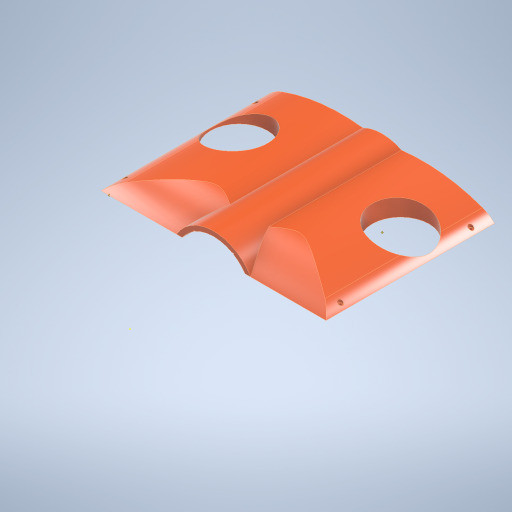
# Autodesk Inventor part: korpus3_gora
Saved by Autodesk Inventor 2024 (Build 280153000, 153)
## iProperties
Created: 2025-05-21
Part Number: korpus3_gora
Material: Tworzywo sztuczne PET
Document SubType Name: Modeling
Designer: Paweł
Density: 1.541 g/cm^3
Appearance: Gładki — jasnopomarańczowy
Mass: 287.612 g
Surface Area: 857.591 cm^2
Volume: 186.64 cm^3
Author: Paweł
Autodesk Inventor part; units mm, degrees
sketch "Szkic1" plane through (0, 0, 0) normal (0, 0, 1) x (1, 0, 0)
  arc A0 (-98.4086, -33.9749) -> (-78.2644, -32.9739) centre (-90, 0) ccw
  arc A1 (119.2902, -19.1594) -> (125, 0) centre (90, 0) ccw
  arc A2 (19.3649, -35) -> (103.6215, -25.7743) centre (42.8262, 140.0954) ccw
  arc A3 (103.6215, -25.7743) -> (125, 0) centre (91.4189, 6.1005) ccw
  line L0 (0, 31.2952) -> (0, 40)
  arc A4 (-103.6215, -25.7743) -> (-19.3649, -35) centre (-42.8262, 140.0954) ccw
  arc A5 (-125, 0) -> (-103.6215, -25.7743) centre (-91.4189, 6.1005) ccw
  arc A6 (-19.3649, 35) -> (-103.6215, 25.7743) centre (-42.8262, -140.0954) ccw
  arc A7 (-103.6215, 25.7743) -> (-125, 0) centre (-91.4189, -6.1005) ccw
  arc A8 (-19.3649, -35) -> (19.3649, -35) centre (0, 0) ccw
  arc A9 (19.3649, 35) -> (-19.3649, 35) centre (0, 0) ccw
  arc A10 (105.3748, -30.457) -> (130.0712, 0) centre (91.4189, 6.1005) ccw
  arc A11 (20.2973, -40.1624) -> (105.3748, -30.457) centre (42.8262, 140.0954) ccw
  arc A12 (-20.2973, -40.1624) -> (20.2973, -40.1624) centre (0, 0) ccw
  arc A13 (-105.3748, -30.457) -> (-20.2973, -40.1624) centre (-42.8262, 140.0954) ccw
  arc A14 (-130.0712, 0) -> (-105.3748, -30.457) centre (-91.4189, 6.1005) ccw
  arc A15 (-105.3748, 30.457) -> (-130.0712, 0) centre (-91.4189, -6.1005) ccw
  arc A16 (-20.2973, 40.1624) -> (-105.3748, 30.457) centre (-42.8262, -140.0954) ccw
  arc A17 (20.2973, 40.1624) -> (-20.2973, 40.1624) centre (0, 0) ccw
  line L1 (0, 0) -> (0, 40)
  arc A18 (103.6215, 25.7743) -> (19.3649, 35) centre (42.8262, -140.0954) ccw
  arc A19 (125, 0) -> (103.6215, 25.7743) centre (91.4189, -6.1005) ccw
  arc A20 (130.0712, 0) -> (105.3748, 30.457) centre (91.4189, -6.1005) ccw
  arc A21 (105.3748, 30.457) -> (20.2973, 40.1624) centre (42.8262, -140.0954) ccw
  point P0 (-119.2902, -19.1594)
  dimension "d1" = 70
  dimension "d2" = 70
  dimension "d4" = 250
  dimension "d6" = 90
  constraints: 46 point on circle, 22 centre point, 10 symmetric about line, 4 end point, 2 horizontal alignment, 1 coincident, 1 collinear, 1 vertical, 13 other
  measures "d1" diameter of A1
  measures "d2" diameter of A0
  measures "d6" distance of point (0, 0) A0.centre
extrude "Wyciągnięcie proste1" add sketch "Szkic1" along normal blind 130 and the other way blind 130
sketch "Szkic2" plane through (0, 0, 130) normal (0, 0, 1) x (1, 0, 0)
  arc A0 (-20.2973, 40.1624) -> (-105.3748, 30.457) centre (-42.8262, -140.0954) ccw projected
  arc A1 (-105.3748, 30.457) -> (-130.0712, 0) centre (-91.4189, -6.1005) ccw projected
  arc A2 (-130.0712, 0) -> (-105.3748, -30.457) centre (-91.4189, 6.1005) ccw projected
  arc A3 (-105.3748, -30.457) -> (-20.2973, -40.1624) centre (-42.8262, 140.0954) ccw projected
  arc A4 (-20.2973, -40.1624) -> (20.2973, -40.1624) centre (0, 0) ccw projected
  arc A5 (20.2973, -40.1624) -> (105.3748, -30.457) centre (42.8262, 140.0954) ccw projected
  arc A6 (105.3748, -30.457) -> (130.0712, 0) centre (91.4189, 6.1005) ccw projected
  arc A7 (130.0712, 0) -> (105.3748, 30.457) centre (91.4189, -6.1005) ccw projected
  arc A8 (105.3748, 30.457) -> (20.2973, 40.1624) centre (42.8262, -140.0954) ccw projected
  arc A9 (20.2973, 40.1624) -> (-20.2973, 40.1624) centre (0, 0) ccw projected
extrude "Wyciągnięcie proste2" add sketch "Szkic2" along normal mid plane 10
sketch "Szkic8" plane through (0, 0, 135) normal (0, 0, 1) x (1, 0, 0)
  circle A0 centre (0, 0) radius 45
  circle A1 centre (0, 0) radius 40
  constraints: 2 centre point, 2 coincident
extrude "Wyciągnięcie proste3" add sketch "Szkic8" along normal blind 70 contours A0 | A1
sketch "Szkic18" plane through (0, 0, 205) normal (0, 0, 1) x (1, 0, 0)
  circle A0 centre (0, 0) radius 45 projected
extrude "Wyciągnięcie proste11" add sketch "Szkic18" along normal blind 5
sketch "Szkic7" plane through (0, 0, 135) normal (0, 0, 1) x (1, 0, 0)
  point P0 (0, 0)
sketch "Szkic10" plane through (0, 0, 205) normal (0, 0, 1) x (1, 0, 0)
  circle A0 centre (0, 0) radius 45 projected
  circle A1 centre (0, 0) radius 40
  dimension "d59" = 5
  constraints: 1 centre point
  measures "d59" radial gap between concentric circles of A0 A1
extrude "Wyciągnięcie proste10" cut sketch "Szkic10" against normal blind 126.25 contours A1
sketch "Szkic12" plane through (0, 0, 0) normal (0, 1, 0) x (-1, 0, 0)
  circle A0 centre (85.2973, -65) radius 32.5
  line L0 (20.2973, -130) -> (20.2973, 135) projected
  line L1 (20.2973, -130) -> (105.3748, -130) projected
  circle A1 centre (-84.3649, -65) radius 32.5
  line L2 (-19.3649, -130) -> (-19.3649, 125) projected
  line L3 (-19.3649, -130) -> (-103.6215, -130) projected
  circle A2 centre (0, 150) radius 32.5
  line L4 (45, 205) -> (-45, 205) projected
  point P0 (0, 0)
  point P1 (-19.3649, 130)
  dimension "d37" = 65
  dimension "d38" = 65
  dimension "d39" = 65
  dimension "d49" = 65
  dimension "d50" = 65
  dimension "d51" = 65
  dimension "d54" = 65
  dimension "d55" = 55
  constraints: 3 centre point
  measures "d37" diameter of A0
  measures "d38" distance from line of L0 A0.centre
  measures "d39" distance from line of L1 A0.centre
  measures "d49" diameter of A1
  measures "d50" distance from line of L2 A1.centre
  measures "d51" distance from line of L3 A1.centre
  measures "d54" diameter of A2
  measures "d55" distance from line of A2.centre L4
extrude "Wyciągnięcie proste6" add sketch "Szkic12" along normal mid plane 111.25
sketch "Szkic33" plane through (84.3649, 55.625, -65) normal (0, 1, 0) x (1, 0, 0)
  circle A0 centre (-84.3649, -215) radius 32.5 projected
  circle A1 centre (0, 0) radius 32.5 projected
  circle A2 centre (-169.6622, 0) radius 32.5 projected
  circle A3 centre (0, 0) radius 30
  circle A4 centre (-169.6622, 0) radius 30
  circle A5 centre (-84.3649, -215) radius 30
  line L0 (-129.3649, -275) -> (-39.3649, -275) projected
  point P0 (-84.3649, -65)
  dimension "d106" = 60
  dimension "d107" = 60
  dimension "d108" = 60
  dimension "d224" = 60
  constraints: 3 centre point, 3 coincident
  measures "d106" diameter of A3
  measures "d107" diameter of A4
  measures "d108" diameter of A5
  measures "d224" distance from line of L0 A0.centre
extrude "Wyciągnięcie proste20" cut sketch "Szkic33" against normal blind 159.75 contours A3 | A4 | A5
sketch "Szkic34" plane through (0, 0, -130) normal (0, 0, -1) x (-1, 0, 0)
  arc A0 (-20.2973, -40.1624) -> (20.2973, -40.1624) centre (0, 0) ccw projected
  arc A1 (20.2973, -40.1624) -> (105.3748, -30.457) centre (42.8262, 140.0954) ccw projected
  arc A2 (105.3748, -30.457) -> (130.0712, 0) centre (91.4189, 6.1005) ccw projected
  arc A3 (130.0712, 0) -> (105.3748, 30.457) centre (91.4189, -6.1005) ccw projected
  arc A4 (105.3748, 30.457) -> (20.2973, 40.1624) centre (42.8262, -140.0954) ccw projected
  arc A5 (20.2973, 40.1624) -> (-20.2973, 40.1624) centre (0, 0) ccw projected
  arc A6 (-20.2973, 40.1624) -> (-105.3748, 30.457) centre (-42.8262, -140.0954) ccw projected
  arc A7 (-105.3748, 30.457) -> (-130.0712, 0) centre (-91.4189, -6.1005) ccw projected
  arc A8 (-130.0712, 0) -> (-105.3748, -30.457) centre (-91.4189, 6.1005) ccw projected
  arc A9 (-105.3748, -30.457) -> (-20.2973, -40.1624) centre (-42.8262, 140.0954) ccw projected
  arc A10 (19.3649, -35) -> (103.6215, -25.7743) centre (42.8262, 140.0954) ccw projected
  arc A11 (-19.3649, -35) -> (19.3649, -35) centre (0, 0) ccw projected
  arc A12 (-103.6215, -25.7743) -> (-19.3649, -35) centre (-42.8262, 140.0954) ccw projected
  arc A13 (-125, 0) -> (-103.6215, -25.7743) centre (-91.4189, 6.1005) ccw projected
  arc A14 (-103.6215, 25.7743) -> (-125, 0) centre (-91.4189, -6.1005) ccw projected
  arc A15 (-19.3649, 35) -> (-103.6215, 25.7743) centre (-42.8262, -140.0954) ccw projected
  arc A16 (19.3649, 35) -> (-19.3649, 35) centre (0, 0) ccw projected
  arc A17 (103.6215, 25.7743) -> (19.3649, 35) centre (42.8262, -140.0954) ccw projected
  arc A18 (125, 0) -> (103.6215, 25.7743) centre (91.4189, -6.1005) ccw projected
  arc A19 (103.6215, -25.7743) -> (125, 0) centre (91.4189, 6.1005) ccw projected
  arc A20 (-27.4304, 93.4644) -> (-123.6952, 79.5576) centre (-42.8262, -140.0954) ccw
  arc A21 (27.4304, 93.4644) -> (-27.4304, 93.4644) centre (0, 0) ccw
  arc A22 (123.6952, 79.5576) -> (27.4304, 93.4644) centre (42.8262, -140.0954) ccw
  arc A23 (182.7526, 0) -> (123.6952, 79.5576) centre (91.4189, -6.1005) ccw
  arc A24 (123.6952, -79.5576) -> (182.7526, 0) centre (91.4189, 6.1005) ccw
  arc A25 (27.4304, -93.4644) -> (123.6952, -79.5576) centre (42.8262, 140.0954) ccw
  arc A26 (-27.4304, -93.4644) -> (27.4304, -93.4644) centre (0, 0) ccw
  arc A27 (-123.6952, -79.5576) -> (-27.4304, -93.4644) centre (-42.8262, 140.0954) ccw
  arc A28 (-182.7526, 0) -> (-123.6952, -79.5576) centre (-91.4189, 6.1005) ccw
  arc A29 (-123.6952, 79.5576) -> (-182.7526, 0) centre (-91.4189, -6.1005) ccw
  constraints: 20 point on circle, 10 centre point, 9 other
extrude "Wyciągnięcie proste21" cut sketch "Szkic34" against normal up to surface (265 mm away) contours A21 A22 A23 A24 A25 A26 A27 A28 A29 A20
sketch "Szkic35" plane through (0, 0, 210) normal (0, 0, 1) x (1, 0, 0)
  circle A0 centre (0, 0) radius 45 projected
  circle A1 centre (0, 0) radius 93.775
  constraints: 1 centre point
extrude "Wyciągnięcie proste22" cut sketch "Szkic35" against normal up to surface (75 mm away)
ref_plane "Płaszczyzna konstrukcyjna8" through (-135.75, 0, 0) normal (1, 0, 0) x (0, 1, 0)
ref_plane "Płaszczyzna konstrukcyjna10" through (-85, 0, 0) normal (1, 0, 0) x (0, 1, 0)
ref_plane "Płaszczyzna konstrukcyjna11" through (-166.25, 0, 0) normal (1, 0, 0) x (0, 1, 0)
sketch "Szkic63" plane through (0, 0, 210) normal (0, 0, 1) x (1, 0, 0)
  circle A0 centre (0, 0) radius 45 projected
extrude "Wyciągnięcie proste37" cut sketch "Szkic63" against normal blind 16.75
ref_plane "Płaszczyzna konstrukcyjna12" through (137, 0, 0) normal (1, 0, 0) x (0, 1, 0)
sketch "Szkic64" plane through (137, 0, 0) normal (1, 0, 0) x (0, 1, 0)
  line L0 (35, -130) -> (35, 123.8992) projected
  line L1 (41.5648, -130) -> (41.5648, 135) projected
  line L2 (0, 135) -> (-30.457, 135) projected
  line L3 (-30.457, 135) -> (-41.5648, 135) projected
  line L4 (41.5648, 135) -> (30.457, 135) projected
  line L5 (30.457, 135) -> (0, 135) projected
  line L6 (2.5, 135) -> (2.5, 125)
  line L7 (-2.5, 135) -> (-2.5, 125)
  line L8 (-41.5648, -130) -> (-41.5648, 135) projected
  line L9 (-30.457, -130) -> (0, -130) projected
  line L10 (0, -130) -> (30.457, -130) projected
  line L11 (36.9405, -94.989) -> (22.5717, -94.989)
  line L12 (41.5648, -0.011) -> (-41.5648, -0.011)
  line L13 (36.9405, -35.011) -> (26.2553, -35.011)
  arc A0 (41.5648, -0.011) -> (22.5717, 47) centre (-46.3041, -8.169) ccw
  arc A1 (2.5, 125) -> (22.5717, 47) centre (167.412, 125.8543) ccw
  line L14 (0, 135) -> (0, -0.011)
  arc A2 (-22.5717, 47) -> (-41.5648, -0.011) centre (46.3041, -8.169) ccw
  arc A3 (-22.5717, 47) -> (-2.5, 125) centre (-167.412, 125.8543) ccw
  line L15 (-2.5, 135) -> (-2.5, 124.9871)
  arc A4 (-2.5, 124.9871) -> (18.3975, 44.2117) centre (167.412, 125.8543) ccw
  arc A5 (35.8963, 4.989) -> (18.3975, 44.2117) centre (-46.3041, -8.169) ccw
  line L16 (35.8963, 4.989) -> (-35.8963, 4.989)
  arc A6 (-18.3975, 44.2117) -> (-35.8963, 4.989) centre (46.3041, -8.169) ccw
  arc A7 (-18.3975, 44.2117) -> (2.5, 124.9871) centre (-167.412, 125.8543) ccw
  line L17 (2.5, 124.9871) -> (2.5, 135)
  line L18 (22.5717, 47) -> (16.9034, 47)
  line L19 (35.8963, 4.989) -> (35.8963, -0.011)
  line L20 (-22.5717, 47) -> (-16.9034, 47)
  line L21 (-35.8963, 4.989) -> (-35.8963, -0.011)
  point P0 (35, 125)
  point P1 (-40.1624, 135)
  point P2 (40.1624, 135)
  point P3 (10.9431, 47)
  dimension "d234" = 10
  dimension "d235" = 10
  dimension "d238" = 35
  dimension "d246" = 5
  constraints: 26 end point, 18 point on circle, 8 centre point, 7 point on line, 4 perpendicular, 3 symmetric about line, 2 horizontal, 2 vertical, 1 midpoint, 11 other
  measures "d234" distance of L6.start L6.end
  measures "d235" distance of L7.start L7.end
  measures "d238" distance between parallel lines of L13 L12
  measures "d246" radial gap between concentric circles of A0 A5
extrude "Wyciągnięcie proste38" cut sketch "Szkic64" against normal up to surface contours A0 A1 L6 L5 L4 L1 | L8 L3 L2 L7 A3 A2 round surface about axis through (0, 0, 0) along (0, 0, 1) radius 45 far side no
ref_plane "Płaszczyzna konstrukcyjna13" through (-136, 0, 0) normal (1, 0, 0) x (0, 1, 0)
sketch "Szkic65" plane through (-136, 0, 0) normal (1, 0, 0) x (0, 1, 0)
  arc A0 (41.5648, 0) -> (22.5717, 47.011) centre (-46.3041, -8.158) ccw
  arc A1 (2.5, 125.011) -> (22.5717, 47.011) centre (167.412, 125.8652) ccw
  arc A2 (-22.5717, 47.011) -> (-2.5, 125.011) centre (-167.412, 125.8652) ccw
  arc A3 (-22.5717, 47.011) -> (-41.5648, 0) centre (46.3041, -8.158) ccw
  line L0 (41.5648, 0) -> (-41.5648, 0)
  line L1 (2.5, 125) -> (2.5, 135) projected
  line L2 (2.5, 125.011) -> (2.5, 135)
  line L3 (2.5, 135) -> (-2.5, 135)
  line L4 (-40.1624, 135) -> (40.1624, 135) projected
  line L5 (-2.5, 125.011) -> (-2.5, 135)
  line L6 (41.5648, 0) -> (41.5648, 135)
  line L7 (41.5648, -130) -> (41.5648, 135) projected
  line L8 (-41.5648, 135) -> (-41.5648, 0)
  line L9 (-45, -130) -> (-45, 193.25) projected
  line L10 (-41.5648, 135) -> (-40.1624, 135)
  line L11 (40.1624, -130) -> (40.1624, 127.9088) projected
  line L12 (41.5648, 135) -> (30.457, 135) projected
  line L13 (40.1624, 135) -> (41.5648, 135)
  arc A4 (-18.6693, 43.8851) -> (-36.5862, -0.4622) centre (46.3041, -8.158) ccw
  arc A5 (36.5862, -0.4622) -> (18.6693, 43.8851) centre (-46.3041, -8.158) ccw
  line L14 (22.5717, 47.011) -> (16.037, 47.011)
  line L15 (-22.5717, 47.011) -> (-16.037, 47.011)
  arc A6 (18.6693, 43.8851) -> (16.037, 47.011) centre (-46.3041, -8.158) ccw
  arc A7 (-16.037, 47.011) -> (-18.6693, 43.8851) centre (46.3041, -8.158) ccw
  point P0 (0, 0)
  point P1 (-22.5717, 47.011)
  point P2 (22.5717, 47.011)
  point P3 (24.9631, 43.8851)
  point P4 (-24.9631, 43.8851)
  point P5 (-36.542, 0)
  point P6 (36.542, 0)
  point P7 (-22.5717, 47.011)
  point P8 (22.5717, 47.011)
  point P9 (-36.7423, 135)
  point P10 (36.7423, 135)
  dimension "d251" = 5
  dimension "d252" = 5
  constraints: 20 end point, 19 point on circle, 8 centre point, 3 horizontal, 3 point on line, 2 collinear, 1 concentric, 1 parallel, 1 perpendicular, 1 vertical
  measures "d251" radial gap between concentric circles of A3 A4
  measures "d252" radial gap between concentric circles of A0 A5
extrude "Wyciągnięcie proste39" cut sketch "Szkic65" along normal up to surface contours A0 A1 L1 L4 L12 L6 | L8 L10 L4 L5 A2 A3 round surface about axis through (0, 0, 0) along (0, 0, 1) radius 45 far side no
sketch "Szkic66" plane through (0, 0, 125) normal (0, 0, -1) x (-1, 0, 0)
  arc A0 (-44.9305, -2.5) -> (-27.1726, -35.8699) centre (0, 0) ccw projected
  arc A1 (-27.1726, -35.8699) -> (-20.7666, -35.1821) centre (-42.8262, 140.0954) ccw projected
  arc A2 (-20.7666, 34.187) -> (-20.7666, -34.187) centre (0, 0) ccw projected
  arc A3 (-20.7666, 35.1821) -> (-27.1726, 35.8699) centre (-42.8262, -140.0954) ccw projected
  arc A4 (-27.1726, 35.8699) -> (-44.9305, 2.5) centre (0, 0) ccw projected
  line L0 (-44.9305, 2.5) -> (-124.4483, 2.5) projected
  arc A5 (-124.4483, 2.5) -> (-125, 0) centre (-91.4189, -6.1005) ccw projected
  arc A6 (-125, 0) -> (-124.4483, -2.5) centre (-91.4189, 6.1005) ccw projected
  line L1 (-124.4483, -2.5) -> (-44.9305, -2.5) projected
  arc A7 (27.1726, -35.8699) -> (44.9305, -2.5001) centre (0, 0) ccw projected
  line L2 (44.9305, -2.5001) -> (124.4482, -2.5001) projected
  arc A8 (124.4482, -2.5001) -> (125, 0) centre (91.4189, 6.1005) ccw projected
  arc A9 (125, 0) -> (124.4482, 2.5001) centre (91.4189, -6.1005) ccw projected
  line L3 (124.4482, 2.5001) -> (44.9305, 2.5001) projected
  arc A10 (44.9305, 2.5001) -> (27.1726, 35.8699) centre (0, 0) ccw projected
  arc A11 (27.1726, 35.8699) -> (20.7666, 35.1821) centre (42.8262, -140.0954) ccw projected
  arc A12 (20.7666, -34.187) -> (20.7666, 34.187) centre (0, 0) ccw projected
  arc A13 (20.7666, -35.1821) -> (27.1726, -35.8699) centre (42.8262, 140.0954) ccw projected
  arc A14 (44.9305, -2.5) -> (44.9305, 2.5) centre (0, 0) ccw projected
  circle A15 centre (0, 0) radius 45
  line L4 (20.7666, 35.1821) -> (20.7666, 34.187) projected
  line L5 (20.7666, -34.187) -> (20.7666, -35.1821) projected
  line L6 (-20.7666, -35.1821) -> (-20.7666, -34.187) projected
  line L7 (-20.7666, 34.187) -> (-20.7666, 35.1821) projected
  point P0 (44.9305, -2.5001)
  point P1 (44.9305, -2.5)
  point P2 (-44.9305, 2.5)
  point P3 (27.1726, 35.8699)
  point P4 (27.1726, -35.8699)
  point P5 (-27.1726, 35.8699)
  point P6 (-27.1726, -35.8699)
  constraints: 1 coincident, 3 other
extrude "Wyciągnięcie proste40" add sketch "Szkic66" along normal blind 105 contours A15 A4 A3 L7 A2 L6 A1 A0 | A13 L5 A12 L4 A11 A10 A14 A7
extrude "Wyciągnięcie proste41" add sketch "Szkic64" against normal up to surface contours L19 A5 L0 A0 L12 | A5 A4 L18 A0 L0 | L12 A2 L20 A7 A6 L21 round surface about axis through (0, 0, 0) along (0, 0, 1) radius 45 far side no
extrude "Wyciągnięcie proste43" add sketch "Szkic65" along normal up to surface contours L0 L11 A0 | L11 L0 A5 A6 L14 A0 | L0 A3 L15 A7 A4 round surface about axis through (0, 0, 0) along (0, 0, 1) radius 45 far side no
ref_plane "Płaszczyzna konstrukcyjna14" through (41.7046, -16.9034, 47) normal (0, 0, 1) x (1, 0, 0)
sketch "Szkic67" plane through (41.7046, -16.9034, 47) normal (0, 0, 1) x (1, 0, 0)
  arc A0 (-21.4073, 57.0658) -> (-24.4603, 58.4682) centre (-41.7046, 16.9034) ccw projected
  arc A1 (-21.4073, 57.0658) -> (-62.0019, 57.0658) centre (-41.7046, 16.9034) ccw projected
  line L0 (-62.0019, 57.0658) -> (-62.0019, 57.0658) projected
  arc A2 (-73.3068, 48.9393) -> (-73.3068, -15.1325) centre (-41.7046, 16.9034) ccw projected
  arc A3 (-62.0019, -23.259) -> (-21.4073, -23.259) centre (-41.7046, 16.9034) ccw projected
  arc A4 (-24.4603, -24.6614) -> (-21.4073, -23.259) centre (-41.7046, 16.9034) ccw projected
  arc A5 (-2.775, -5.6684) -> (0, 0) centre (-41.7046, 16.9034) ccw projected
  arc A6 (-10.0984, -15.1286) -> (-10.0984, 48.9354) centre (-41.7046, 16.9034) ccw projected
  arc A7 (0, 33.8068) -> (-2.775, 39.4751) centre (-41.7046, 16.9034) ccw projected
  line L1 (-86.6351, 19.4034) -> (-86.6351, 19.4034) projected
  arc A8 (-86.6351, 19.4034) -> (-86.6351, 14.4034) centre (-41.7046, 16.9034) ccw projected
  line L2 (-86.6351, 14.4033) -> (-86.6351, 14.4034) projected
  arc A9 (-86.6351, 19.4034) -> (-86.6351, 14.4033) centre (-41.7046, 16.9034) ccw projected
  arc A10 (3.2259, 14.4034) -> (3.2259, 19.4034) centre (-41.7046, 16.9034) ccw projected
  arc A11 (3.2259, 14.4034) -> (3.2259, 19.4034) centre (-41.7046, 16.9034) ccw projected
  circle A12 centre (-41.7046, 16.9034) radius 45 projected
  line L3 (74.9279, 0) -> (0, 0) projected
  line L4 (74.9279, 33.8068) -> (0, 33.8068) projected
  line L5 (68.2294, 39.4751) -> (-2.775, 39.4751) projected
  line L6 (68.2294, -5.6684) -> (-2.775, -5.6684) projected
  spline S0 degree 8 poles (61.9169, -8.8709) (63.6085, -8.2233) (65.223, -7.4876) (66.7628, -6.6721) (68.2309, -5.7826) (69.6315, -4.8225) (70.9701, -3.7914) (72.2516, -2.6847) (73.4789, -1.4941) knots 0 0 0 0 0 0 0 0 0 1 1 1 1 1 1 1 1 1 projected
  spline S1 degree 4 poles (73.4789, -1.4941) (73.8652, -1.1194) (74.2349, -0.745) (74.5889, -0.3716) (74.9279, 0) knots 0 0 0 0 0 1 1 1 1 1 projected
  arc A13 (68.2294, -5.6684) -> (74.9279, 0) centre (49.7143, 23.0038) ccw projected
  spline S2 degree 8 poles (68.2294, -5.6684) (69.6364, -4.7598) (70.9108, -3.825) (72.0633, -2.8799) (73.1046, -1.9365) (74.0451, -1.0038) (74.8947, -0.0887) (75.6624, 0.804) (77.0847, 2.5803) (77.7326, 3.4621) (78.3092, 4.312) (78.8227, 5.127) (79.2802, 5.9055) (79.6881, 6.6464) (80.0521, 7.3492) (81.142, 9.5785) (81.6905, 10.9319) (82.0822, 12.0632) (82.3584, 12.9712) (82.5486, 13.6577) (82.6712, 14.1252) (82.736, 14.3742) (82.7436, 14.4034) knots 0 0 0 0 0 0 0 0 0 0.221338 0.221338 0.221338 0.221338 0.221338 0.221338 0.221338 0.453504 0.453504 0.453504 0.453504 0.453504 0.453504 0.453504 1 1 1 1 1 1 1 1 1 projected
  arc A14 (82.7436, 14.4034) -> (83.2954, 16.9034) centre (49.7143, 23.0038) ccw projected
  arc A15 (61.9169, -8.8709) -> (83.2954, 16.9034) centre (49.7143, 23.0038) ccw projected
  arc A16 (74.9279, 33.8068) -> (68.2294, 39.4751) centre (49.7143, 10.8029) ccw projected
  arc A17 (83.2954, 16.9034) -> (61.9169, 42.6777) centre (49.7143, 10.8029) ccw projected
  arc A18 (83.2954, 16.9034) -> (82.7436, 19.4034) centre (49.7143, 10.8029) ccw projected
  arc A19 (-62.0019, -23.259) -> (-58.9489, -24.6614) centre (-41.7046, 16.9034) ccw projected
  arc A20 (-58.9489, 58.4682) -> (-62.0019, 57.0658) centre (-41.7046, 16.9034) ccw projected
  arc A21 (-79.1458, 41.8665) -> (-82.6492, 35.5727) centre (-41.7046, 16.9034) ccw projected
  arc A22 (-82.6492, -1.7659) -> (-79.1458, -8.0597) centre (-41.7046, 16.9034) ccw projected
  arc A23 (-156.6047, -1.7659) -> (-147.2643, -8.0597) centre (-133.1235, 23.0038) ccw projected
  line L7 (-147.2643, -8.0597) -> (-79.1458, -8.0597) projected
  arc A24 (-82.6492, -1.7659) -> (-79.1458, -8.0597) centre (-41.7046, 16.9034) ccw projected
  line L8 (-156.6047, -1.7659) -> (-82.6492, -1.7659) projected
  arc A25 (-147.2643, 41.8665) -> (-156.6047, 35.5727) centre (-133.1235, 10.8029) ccw
  line L9 (-156.6047, 35.5727) -> (-82.6492, 35.5727)
  arc A26 (-79.1458, 41.8665) -> (-82.6492, 35.5727) centre (-41.7046, 16.9034) ccw
  line L10 (-147.2643, 41.8665) -> (-79.1458, 41.8665)
  arc A27 (-62.0019, -23.259) -> (-58.9489, -24.6614) centre (-41.7046, 16.9034) ccw projected
  arc A28 (-62.0019, -23.259) -> (-21.4073, -23.259) centre (-41.7046, 16.9034) ccw projected
  arc A29 (-24.4603, -24.6614) -> (-21.4073, -23.259) centre (-41.7046, 16.9034) ccw projected
  arc A30 (-2.775, -5.6684) -> (0, 0) centre (-41.7046, 16.9034) ccw projected
  arc A31 (-10.0984, -15.1286) -> (-10.0984, 48.9354) centre (-41.7046, 16.9034) ccw projected
  arc A32 (0, 33.8068) -> (-2.775, 39.4751) centre (-41.7046, 16.9034) ccw projected
  arc A33 (-21.4073, 57.0658) -> (-24.4603, 58.4682) centre (-41.7046, 16.9034) ccw projected
  arc A34 (-21.4073, 57.0658) -> (-62.0019, 57.0658) centre (-41.7046, 16.9034) ccw projected
  arc A35 (-58.9489, 58.4682) -> (-62.0019, 57.0658) centre (-41.7046, 16.9034) ccw projected
  arc A36 (-79.1458, 41.8665) -> (-82.6492, 35.5727) centre (-41.7046, 16.9034) ccw projected
  arc A37 (-73.3068, 48.9393) -> (-73.3068, -15.1325) centre (-41.7046, 16.9034) ccw projected
  arc A38 (-82.6492, -1.7659) -> (-79.1458, -8.0597) centre (-41.7046, 16.9034) ccw projected
  line L11 (-86.6351, 19.4034) -> (-86.6351, 19.4034) projected
  arc A39 (-86.6351, 19.4034) -> (-86.6351, 14.4034) centre (-41.7046, 16.9034) ccw projected
  line L12 (-86.6351, 14.4033) -> (-86.6351, 14.4034) projected
  arc A40 (-86.6351, 19.4034) -> (-86.6351, 14.4033) centre (-41.7046, 16.9034) ccw projected
  arc A41 (3.2259, 14.4034) -> (3.2259, 19.4034) centre (-41.7046, 16.9034) ccw projected
  arc A42 (3.2259, 14.4034) -> (3.2259, 19.4034) centre (-41.7046, 16.9034) ccw projected
  circle A43 centre (-41.7046, 16.9034) radius 45 projected
  arc A44 (-166.7046, 16.9034) -> (-145.3261, -8.8709) centre (-133.1235, 23.0038) ccw projected
  arc A45 (-145.3261, 42.6777) -> (-166.7046, 16.9034) centre (-133.1235, 10.8029) ccw projected
  arc A46 (-151.6387, 39.4751) -> (-159.1012, 32.9404) centre (-133.1235, 10.8029) ccw projected
  arc A47 (-166.1529, 19.4034) -> (-166.7046, 16.9034) centre (-133.1235, 10.8029) ccw projected
  arc A48 (-159.1012, 0.8664) -> (-151.6387, -5.6684) centre (-133.1235, 23.0038) ccw projected
  arc A49 (-166.7046, 16.9034) -> (-166.1529, 14.4033) centre (-133.1235, 23.0038) ccw projected
  arc A50 (-159.1012, 0.8664) -> (-151.6387, -5.6684) centre (-133.1235, 23.0038) ccw projected
  line L13 (-151.6387, -5.6684) -> (-80.6343, -5.6684) projected
  arc A51 (-83.75, 0.8664) -> (-80.6343, -5.6684) centre (-41.7046, 16.9034) ccw projected
  line L14 (-159.1012, 0.8664) -> (-83.75, 0.8664) projected
  line L15 (-159.1012, 32.9404) -> (-83.75, 32.9404) projected
  arc A52 (-151.6387, 39.4751) -> (-159.1012, 32.9404) centre (-133.1235, 10.8029) ccw projected
  line L16 (-159.1012, 32.9404) -> (-83.75, 32.9404) projected
  arc A53 (-80.6343, 39.4751) -> (-83.75, 32.9404) centre (-41.7046, 16.9034) ccw projected
  line L17 (-151.6387, 39.4751) -> (-80.6343, 39.4751) projected
  point P0 (-2.775, 39.4751)
  point P1 (0, 0)
  point P2 (74.7546, -0.1886)
  point P3 (83.2954, 16.9034)
  point P4 (-156.6047, 35.5727)
  point P5 (-156.6047, -1.7659)
  point P6 (-151.6387, -5.6684)
  point P7 (-80.6343, -5.6684)
  constraints: 4 horizontal alignment, 2 centre point, 2 end point, 46 other
extrude "Wyciągnięcie proste42" add sketch "Szkic67" against normal blind 5 contours L5 A16 L4 A6 | L4 A17 A14 S2 L3 A6 | A2 L9 A25 L17 | A2 L15 A45 L9 | L3 S1 S0 L6 A5 | A2 L14 A44 A45 L15 | A2 L8 A44 L14 | A2 L13 A23 L8
sketch "Szkic68" plane through (0, 0, -130) normal (0, 0, -1) x (-1, 0, 0)
  arc A0 (-20.2973, -40.1624) -> (20.2973, -40.1624) centre (0, 0) ccw projected
  arc A1 (20.2973, -40.1624) -> (105.3748, -30.457) centre (42.8262, 140.0954) ccw projected
  arc A2 (105.3748, -30.457) -> (130.0712, 0) centre (91.4189, 6.1005) ccw projected
  arc A3 (130.0712, 0) -> (105.3748, 30.457) centre (91.4189, -6.1005) ccw projected
  arc A4 (105.3748, 30.457) -> (20.2973, 40.1624) centre (42.8262, -140.0954) ccw projected
  arc A5 (20.2973, 40.1624) -> (-20.2973, 40.1624) centre (0, 0) ccw projected
  arc A6 (-20.2973, 40.1624) -> (-105.3748, 30.457) centre (-42.8262, -140.0954) ccw projected
  arc A7 (-105.3748, 30.457) -> (-130.0712, 0) centre (-91.4189, -6.1005) ccw projected
  arc A8 (-130.0712, 0) -> (-105.3748, -30.457) centre (-91.4189, 6.1005) ccw projected
  arc A9 (-105.3748, -30.457) -> (-20.2973, -40.1624) centre (-42.8262, 140.0954) ccw projected
  arc A10 (19.3649, -35) -> (103.6215, -25.7743) centre (42.8262, 140.0954) ccw projected
  arc A11 (-19.3649, -35) -> (19.3649, -35) centre (0, 0) ccw projected
  arc A12 (-103.6215, -25.7743) -> (-19.3649, -35) centre (-42.8262, 140.0954) ccw projected
  arc A13 (-125, 0) -> (-103.6215, -25.7743) centre (-91.4189, 6.1005) ccw projected
  arc A14 (-103.6215, 25.7743) -> (-125, 0) centre (-91.4189, -6.1005) ccw projected
  arc A15 (-19.3649, 35) -> (-103.6215, 25.7743) centre (-42.8262, -140.0954) ccw projected
  arc A16 (19.3649, 35) -> (-19.3649, 35) centre (0, 0) ccw projected
  arc A17 (103.6215, 25.7743) -> (19.3649, 35) centre (42.8262, -140.0954) ccw projected
  arc A18 (125, 0) -> (103.6215, 25.7743) centre (91.4189, -6.1005) ccw projected
  arc A19 (103.6215, -25.7743) -> (125, 0) centre (91.4189, 6.1005) ccw projected
  arc A20 (-28.1786, 100.3599) -> (-126.0804, 85.9622) centre (-42.8262, -140.0954) ccw
  arc A21 (28.1786, 100.3599) -> (-28.1786, 100.3599) centre (0, 0) ccw
  arc A22 (126.0804, 85.9622) -> (28.1786, 100.3599) centre (42.8262, -140.0954) ccw
  arc A23 (189.6011, 0) -> (126.0804, 85.9622) centre (91.4189, -6.1005) ccw
  arc A24 (126.0804, -85.9622) -> (189.6011, 0) centre (91.4189, 6.1005) ccw
  arc A25 (28.1786, -100.3599) -> (126.0804, -85.9622) centre (42.8262, 140.0954) ccw
  arc A26 (-28.1786, -100.3599) -> (28.1786, -100.3599) centre (0, 0) ccw
  arc A27 (-126.0804, -85.9622) -> (-28.1786, -100.3599) centre (-42.8262, 140.0954) ccw
  arc A28 (-189.6011, 0) -> (-126.0804, -85.9622) centre (-91.4189, 6.1005) ccw
  arc A29 (-126.0804, 85.9622) -> (-189.6011, 0) centre (-91.4189, -6.1005) ccw
  constraints: 20 point on circle, 10 centre point, 9 other
extrude "Wyciągnięcie proste44" cut sketch "Szkic68" against normal blind 393 contours A21 A22 A23 A24 A25 A26 A27 A28 A29 A20
sketch "Szkic69" plane through (0, 0, 125) normal (0, 0, -1) x (-1, 0, 0)
  line L0 (-44.9305, 2.5) -> (-124.4483, 2.5) projected
  arc A0 (-124.4483, 2.5) -> (-125, 0) centre (-91.4189, -6.1005) ccw projected
  arc A1 (-125, 0) -> (-124.4483, -2.5) centre (-91.4189, 6.1005) ccw projected
  line L1 (-124.4483, -2.5) -> (-44.9305, -2.5) projected
  line L2 (44.9305, -2.5001) -> (124.4482, -2.5001) projected
  arc A2 (124.4482, -2.5001) -> (125, 0) centre (91.4189, 6.1005) ccw projected
  arc A3 (125, 0) -> (124.4482, 2.5001) centre (91.4189, -6.1005) ccw projected
  line L3 (124.4482, 2.5001) -> (44.9305, 2.5001) projected
  arc A4 (-44.9305, 2.5) -> (-44.9305, -2.5) centre (0, 0) ccw projected
  arc A5 (44.9305, -2.5001) -> (44.9305, 2.5001) centre (0, 0) ccw projected
extrude "Wyciągnięcie proste45" add sketch "Szkic69" along normal blind 10
fillet "Zaokrąglenie10" radius 2 2 edges at (-84.6894, 2.5001, 115) (-84.6894, -2.5001, 115)
fillet "Zaokrąglenie11" radius 2 2 edges at (84.6894, 2.5, 115) (84.6894, -2.5, 115)
sketch "Szkic70" plane through (0, 0, 135) normal (0, 0, 1) x (1, 0, 0)
  line L0 (44.9305, -2.5) -> (129.5928, -2.5) projected
  arc A0 (129.5928, -2.5) -> (130.0712, 0) centre (91.4189, 6.1005) ccw projected
  arc A1 (130.0712, 0) -> (129.5928, 2.5) centre (91.4189, -6.1005) ccw projected
  line L1 (129.5928, 2.5) -> (44.9305, 2.5) projected
  arc A2 (44.9305, -2.5) -> (44.9305, 2.5) centre (0, 0) ccw projected
  line L2 (-129.5928, -2.5) -> (-44.9305, -2.5) projected
  arc A3 (-44.9305, 2.5) -> (-44.9305, -2.5) centre (0, 0) ccw projected
  line L3 (-44.9305, 2.5) -> (-129.5928, 2.5) projected
  arc A4 (-129.5928, 2.5) -> (-130.0712, 0) centre (-91.4189, -6.1005) ccw projected
  arc A5 (-130.0712, 0) -> (-129.5928, -2.5) centre (-91.4189, 6.1005) ccw projected
extrude "Wyciągnięcie proste46" add sketch "Szkic70" along normal blind 40
sketch "Szkic71" plane through (38.9296, 22.5717, 47) normal (0, 0, 1) x (1, 0, 0)
  line L0 (46.0981, -25.7813) -> (53.0981, -25.7813)
  arc A0 (53.0981, -25.7813) -> (53.0981, -19.7813) centre (53.0981, -22.7813) ccw
  line L1 (53.0981, -19.7813) -> (46.0981, -19.7813)
  arc A1 (39.0981, -12.7813) -> (46.0981, -19.7813) centre (46.0981, -12.7813) ccw
  line L2 (39.0981, -12.7813) -> (39.0981, -5.7813)
  arc A2 (39.0981, -5.7813) -> (33.0981, -5.7813) centre (36.0981, -5.7813) ccw
  line L3 (33.0981, -5.7813) -> (33.0981, -12.7813)
  arc A3 (26.0981, -19.7813) -> (33.0981, -12.7813) centre (26.0981, -12.7813) ccw
  line L4 (26.0981, -19.7813) -> (19.0981, -19.7813)
  arc A4 (19.0981, -19.7813) -> (19.0981, -25.7813) centre (19.0981, -22.7813) ccw
  line L5 (19.0981, -25.7813) -> (26.0981, -25.7813)
  arc A5 (33.0981, -32.7813) -> (26.0981, -25.7813) centre (26.0981, -32.7813) ccw
  line L6 (33.0981, -32.7813) -> (33.0981, -39.7813)
  arc A6 (33.0981, -39.7813) -> (39.0981, -39.7813) centre (36.0981, -39.7813) ccw
  line L7 (39.0981, -39.7813) -> (39.0981, -32.7813)
  arc A7 (46.0981, -25.7813) -> (39.0981, -32.7813) centre (46.0981, -32.7813) ccw
  circle A8 centre (36.0981, -5.7813) radius 1.5
  circle A9 centre (53.0981, -22.7813) radius 1.5
  circle A10 centre (36.0981, -39.7813) radius 1.5
  circle A11 centre (19.0981, -22.7813) radius 1.5
  circle A12 centre (36.0984, -22.7813) radius 3.9995
  arc A13 (0, -45.1435) -> (0, 0) centre (-38.9296, -22.5717) ccw projected
  circle A14 centre (-38.9296, -22.5717) radius 40 projected
  line L8 (-38.9296, -22.5717) -> (-38.9296, 15.8683)
  arc A15 (-103.9574, -25.7813) -> (-110.9574, -32.7813) centre (-103.9574, -32.7813) ccw
  line L9 (-103.9574, -19.7813) -> (-96.9574, -19.7813)
  line L10 (-96.9574, -25.7813) -> (-103.9574, -25.7813)
  circle A16 centre (-96.9574, -22.7813) radius 1.5
  arc A17 (-96.9574, -25.7813) -> (-96.9574, -19.7813) centre (-96.9574, -22.7813) ccw
  circle A18 centre (-113.9574, -39.7813) radius 1.5
  line L11 (-116.9574, -39.7813) -> (-116.9574, -32.7813)
  arc A19 (-116.9574, -32.7813) -> (-123.9574, -25.7813) centre (-123.9574, -32.7813) ccw
  line L12 (-130.9574, -19.7813) -> (-123.9574, -19.7813)
  arc A20 (-130.9574, -19.7813) -> (-130.9574, -25.7813) centre (-130.9574, -22.7813) ccw
  circle A21 centre (-130.9574, -22.7813) radius 1.5
  line L13 (-123.9574, -25.7813) -> (-130.9574, -25.7813)
  arc A22 (-116.9574, -39.7813) -> (-110.9574, -39.7813) centre (-113.9574, -39.7813) ccw
  line L14 (-110.9574, -32.7813) -> (-110.9574, -39.7813)
  arc A23 (-123.9574, -19.7813) -> (-116.9574, -12.7813) centre (-123.9574, -12.7813) ccw
  line L15 (-116.9574, -12.7813) -> (-116.9574, -5.7813)
  arc A24 (-110.9574, -12.7813) -> (-103.9574, -19.7813) centre (-103.9574, -12.7813) ccw
  line L16 (-110.9574, -5.7813) -> (-110.9574, -12.7813)
  arc A25 (-110.9574, -5.7813) -> (-116.9574, -5.7813) centre (-113.9574, -5.7813) ccw
  circle A26 centre (-113.9574, -5.7813) radius 1.5
  circle A27 centre (-113.9576, -22.7813) radius 3.9995
  arc A28 (-77.8593, 0) -> (-77.8593, -45.1435) centre (-38.9296, -22.5717) ccw
  circle A29 centre (-38.9296, -22.5717) radius 40
  point P0 (-38.9296, -22.5717)
  point P1 (6.0704, -22.5717)
  point P2 (6.0704, -22.5717)
  point P3 (-83.9296, -22.5717)
  point P4 (-83.9296, -22.5717)
  constraints: 36 point on circle, 34 end point, 34 symmetric about line, 28 centre point, 2 coincident, 1 vertical, 15 other
extrude "Wyciągnięcie proste47" cut sketch "Szkic71" against normal blind 40 contours A8 | A9 | A10 | A11 | A16 | A18 | A21 | A26
sketch "Szkic72" plane through (-117.3966, 16.037, 47.011) normal (0, 0, 1) x (1, 0, 0)
  arc A0 (0, -32.074) -> (7.4625, -38.6087) centre (25.9776, -9.9365) ccw projected
  line L0 (7.4625, -38.6087) -> (78.4669, -38.6087) projected
  arc A1 (75.3512, -32.074) -> (78.4669, -38.6087) centre (117.3966, -16.037) ccw projected
  line L1 (0, -32.074) -> (75.3512, -32.074) projected
  arc A2 (7.4625, 6.5347) -> (0, 0) centre (25.9776, -22.1375) ccw projected
  line L2 (0, 0) -> (75.3512, 0) projected
  arc A3 (78.4669, 6.5347) -> (75.3512, 0) centre (117.3966, -16.037) ccw projected
  line L3 (7.4625, 6.5347) -> (78.4669, 6.5347) projected
extrude "Wyciągnięcie proste48" cut sketch "Szkic72" against normal blind 0.1
sketch "Szkic73" plane through (0, 0, -130) normal (0, 0, -1) x (-1, 0, 0)
  arc A0 (-103.6215, 25.7743) -> (-125, 0) centre (-91.4189, -6.1005) ccw projected
  circle A1 centre (-125, 0) radius 5
  arc A2 (-130.0712, 0) -> (-105.3748, -30.457) centre (-91.4189, 6.1005) ccw projected
  circle A3 centre (-125, 0) radius 1.5
  arc A4 (125, 0) -> (117.3966, 16.037) centre (91.4189, -6.1005) ccw projected
  circle A5 centre (125, 0) radius 5
  arc A6 (105.3748, -30.457) -> (130.0712, 0) centre (91.4189, 6.1005) ccw projected
  circle A7 centre (125, 0) radius 1.5
  point P0 (0, 0)
  dimension "d275" = 3
  dimension "d276" = 3
  constraints: 4 centre point, 2 coincident, 2 tangent
  measures "d275" diameter of A3
  measures "d276" diameter of A7
extrude "Wyciągnięcie proste49" add sketch "Szkic73" against normal blind 10 contours A1 | A3 | A5
sketch "Szkic74" plane through (0, 0, -130) normal (0, 0, -1) x (-1, 0, 0)
  arc A0 (-113.2597, 20.1271) -> (-125, 0) centre (-91.4189, -6.1005) ccw projected
  circle A1 centre (-125, 0) radius 1.5
  arc A2 (123.7484, 4.8408) -> (123.7484, -4.8408) centre (125, 0) ccw projected
  arc A3 (125, 0) -> (124.6995, 1.4696) centre (91.4189, -6.1005) ccw projected
  circle A4 centre (125, 0) radius 1.5
  point P0 (0, 0)
  dimension "d279" = 3
  constraints: 1 centre point, 1 coincident, 3 other
  measures "d279" diameter of A1
extrude "Wyciągnięcie proste50" cut sketch "Szkic74" against normal blind 10
ref_plane "Płaszczyzna konstrukcyjna15" through (0, -45, -130) normal (0, 1, 0) x (-1, 0, 0)
sketch "Szkic75" plane through (0, -45, -130) normal (0, 1, 0) x (-1, 0, 0)
  line L0 (-50, 10) -> (50, 10)
  line L1 (50, 10) -> (50, 110)
  line L2 (50, 110) -> (-50, 110)
  line L3 (-50, 110) -> (-50, 10)
  line L4 (-20.2973, 0) -> (20.2973, 0) projected
  point P0 (0, 130)
  point P1 (0, 10)
  point P2 (0, 0)
  dimension "d283" = 100
  dimension "d284" = 100
  dimension "d285" = 10
  constraints: 8 end point, 2 midpoint, 2 parallel, 1 horizontal, 1 perpendicular, 1 vertical alignment
  measures "d283" distance of L0.start L0.end
  measures "d284" distance of L2.end L0.start
  measures "d285" distance from line of point (0, 0) L0
extrude "Wyciągnięcie proste51" add sketch "Szkic75" along normal blind 4
sketch "Szkic76" plane through (0, 0, 193.25) normal (0, 0, 1) x (1, 0, 0)
  circle A0 centre (0, 0) radius 45
  constraints: 1 centre point, 1 coincident
extrude "Wyciągnięcie proste52" add sketch "Szkic76" against normal blind 5
sketch "Szkic77" plane through (0, -45, -130) normal (0, -1, 0) x (1, 0, 0)
  line L0 (-50, 110) -> (0, 110) projected
  line L1 (-50, 10) -> (-50, 110) projected
  line L2 (0, 10) -> (-50, 10) projected
  line L3 (50, 10) -> (0, 10) projected
  line L4 (50, 110) -> (50, 10) projected
  line L5 (0, 110) -> (50, 110) projected
  point P0 (0, 130)
extrude "Wyciągnięcie proste53" add sketch "Szkic77" along normal blind 1
sketch "Szkic78" plane through (0, 0, -130) normal (0, 0, -1) x (-1, 0, 0)
  arc A0 (123.7484, 4.8408) -> (123.7484, -4.8408) centre (125, 0) ccw projected
  circle A1 centre (125, 0) radius 5
  point P0 (0, 0)
  constraints: 1 centre point, 1 coincident
sketch "Szkic79" plane through (0, 0, -130) normal (0, 0, -1) x (-1, 0, 0)
  arc A0 (105.3748, -30.457) -> (130.0712, 0) centre (91.4189, 6.1005) ccw projected
  arc A1 (130.0712, 0) -> (105.3748, 30.457) centre (91.4189, -6.1005) ccw projected
  arc A2 (105.3748, 30.457) -> (20.2973, 40.1624) centre (42.8262, -140.0954) ccw projected
  arc A3 (20.2973, 40.1624) -> (-20.2973, 40.1624) centre (0, 0) ccw projected
  arc A4 (-20.2973, 40.1624) -> (-105.3748, 30.457) centre (-42.8262, -140.0954) ccw projected
  arc A5 (-105.3748, 30.457) -> (-130.0712, 0) centre (-91.4189, -6.1005) ccw projected
  arc A6 (-130.0712, 0) -> (-105.3748, -30.457) centre (-91.4189, 6.1005) ccw projected
  arc A7 (-105.3748, -30.457) -> (-20.2973, -40.1624) centre (-42.8262, 140.0954) ccw projected
  arc A8 (-20.2973, -40.1624) -> (20.2973, -40.1624) centre (0, 0) ccw projected
  arc A9 (20.2973, -40.1624) -> (105.3748, -30.457) centre (42.8262, 140.0954) ccw projected
  circle A10 centre (125, 0) radius 1.5 projected
  arc A11 (103.6215, -25.7743) -> (123.7484, -4.8408) centre (91.4189, 6.1005) ccw projected
  arc A12 (19.3649, -35) -> (103.6215, -25.7743) centre (42.8262, 140.0954) ccw projected
  arc A13 (-19.3649, -35) -> (19.3649, -35) centre (0, 0) ccw projected
  arc A14 (-103.6215, -25.7743) -> (-19.3649, -35) centre (-42.8262, 140.0954) ccw projected
  arc A15 (-123.7484, -4.8408) -> (-103.6215, -25.7743) centre (-91.4189, 6.1005) ccw projected
  arc A16 (-123.7484, -4.8408) -> (-123.7484, 4.8408) centre (-125, 0) ccw projected
  arc A17 (-103.6215, 25.7743) -> (-123.7484, 4.8408) centre (-91.4189, -6.1005) ccw projected
  arc A18 (-19.3649, 35) -> (-103.6215, 25.7743) centre (-42.8262, -140.0954) ccw projected
  arc A19 (19.3649, 35) -> (-19.3649, 35) centre (0, 0) ccw projected
  arc A20 (103.6215, 25.7743) -> (19.3649, 35) centre (42.8262, -140.0954) ccw projected
  arc A21 (123.7484, 4.8408) -> (103.6215, 25.7743) centre (91.4189, -6.1005) ccw projected
  arc A22 (123.7484, 4.8408) -> (123.7484, -4.8408) centre (125, 0) ccw projected
  circle A23 centre (-125, 0) radius 1.5 projected
  arc A24 (19.7476, 37.0679) -> (-19.7476, 37.0679) centre (0, 0) ccw
  arc A25 (-19.7476, 37.0679) -> (-104.323, 27.6473) centre (-42.8262, -140.0954) ccw
  arc A26 (-104.323, 27.6473) -> (-126.4847, 2.6068) centre (-91.4189, -6.1005) ccw
  arc A27 (-126.4847, -2.6068) -> (-104.323, -27.6473) centre (-91.4189, 6.1005) ccw
  arc A28 (-104.323, -27.6473) -> (-19.7476, -37.0679) centre (-42.8262, 140.0954) ccw
  arc A29 (-19.7476, -37.0679) -> (19.7476, -37.0679) centre (0, 0) ccw
  arc A30 (19.7476, -37.0679) -> (104.323, -27.6473) centre (42.8262, 140.0954) ccw
  arc A31 (104.323, -27.6473) -> (126.4847, -2.6068) centre (91.4189, 6.1005) ccw
  arc A32 (126.4847, 2.6068) -> (104.323, 27.6473) centre (91.4189, -6.1005) ccw
  arc A33 (104.323, 27.6473) -> (19.7476, 37.0679) centre (42.8262, -140.0954) ccw
  arc A34 (-123.7484, 4.8408) -> (-124.6995, 1.4696) centre (-91.4189, -6.1005) ccw projected
  arc A35 (-124.6995, -1.4696) -> (-123.7484, -4.8408) centre (-91.4189, 6.1005) ccw projected
  arc A36 (-125.6428, 5.4819) -> (-126.6497, 1.9132) centre (-91.4189, -6.1005) ccw
  arc A37 (-126.6497, -1.9132) -> (-125.6428, -5.4819) centre (-91.4189, 6.1005) ccw
  arc A38 (-127.0309, 0) -> (-126.6497, -1.9132) centre (-91.4189, 6.1005) ccw
  arc A39 (-126.6497, 1.9132) -> (-127.0309, 0) centre (-91.4189, -6.1005) ccw
  arc A40 (127.0309, 0) -> (126.4847, 2.6068) centre (91.4189, -6.1005) ccw
  arc A41 (126.4847, -2.6068) -> (127.0309, 0) centre (91.4189, 6.1005) ccw
  point P0 (-126.4847, 2.6068)
  point P1 (-126.4847, -2.6068)
  dimension "d292" = 2
  constraints: 32 point on circle, 16 centre point, 7 other
  measures "d292" radial gap between concentric circles of A20 A33
extrude "Wyciągnięcie proste54" cut sketch "Szkic79" against normal blind 2 contours A35 A23 A34 A16 | A33 A32 A40 A41 A31 A30 A29 A28 A27 A37 A38 A39 A36 A26 A25 A24
ref_plane "Płaszczyzna konstrukcyjna17" through (0, 47.25, 0) normal (0, 1, 0) x (-1, 0, 0)
ref_plane "Płaszczyzna konstrukcyjna18" through (38.9296, 22.5717, 44.5) normal (0, 0, 1) x (1, 0, 0)
ref_plane "Płaszczyzna konstrukcyjna21" through (-109.934, 22.5717, 47.011) normal (0, 0, 1) x (1, 0, 0)
sketch "Szkic83" plane through (-109.934, 22.5717, 47.011) normal (0, 0, 1) x (1, 0, 0)
  line L0 (-29.7359, 25.5294) -> (246.7356, 25.5294)
  line L1 (246.7356, 25.5294) -> (246.7356, -73.1)
  line L2 (246.7356, -73.1) -> (-29.7359, -73.1)
  line L3 (-29.7359, -73.1) -> (-29.7359, 25.5294)
  point P0 (109.934, -22.5717)
  constraints: 8 end point, 2 parallel, 1 horizontal, 1 perpendicular
extrude "Wyciągnięcie proste57" cut sketch "Szkic83" along normal blind 190
ref_plane "Płaszczyzna konstrukcyjna22" through (-109.934, 22.5717, 47.011) normal (0, 1, 0) x (-1, 0, 0)
sketch "Szkic84" plane through (-109.934, 22.5717, 47.011) normal (0, 1, 0) x (-1, 0, 0)
  line L0 (-248.2049, -185.912) -> (28.8357, -185.912)
  line L1 (28.8357, -185.912) -> (28.8357, 15.0088)
  line L2 (28.8357, 15.0088) -> (-248.2049, 15.0088)
  line L3 (-248.2049, 15.0088) -> (-248.2049, -185.912)
  point P0 (-109.934, -47.011)
  constraints: 8 end point, 2 parallel, 1 horizontal, 1 perpendicular
extrude "Wyciągnięcie proste58" cut sketch "Szkic84" against normal blind 190
sketch "Szkic85" plane through (-109.934, 22.5717, 38.5983) normal (0, -1, 0) x (1, 0, 0)
  circle A0 centre (-3.1141, -148.5983) radius 1.5
  circle A1 centre (222.8859, -11.5983) radius 1.5
  circle A2 centre (-3.1141, -11.5983) radius 1.5
  circle A3 centre (222.8859, -148.5983) radius 1.5
  circle A4 centre (222.8859, -11.5983) radius 5
  circle A5 centre (-3.1141, -11.5983) radius 5
  circle A6 centre (222.8859, -148.5983) radius 5
  circle A7 centre (-3.1141, -148.5983) radius 5
  line L0 (302.8766, 39.7263) -> (307.521, 39.7263)
  line L1 (228.4025, -137.2847) -> (299.4069, -137.2847)
  line L2 (5.611, -168.5983) -> (-3.4697, -168.5983) projected
  line L3 (-8.1141, -168.5983) -> (-8.1141, 8.4127) projected
  line L4 (227.9822, 8.4017) -> (227.9822, -168.5983) projected
  line L5 (227.9822, 8.4017) -> (148.8637, 8.4017) projected
  point P0 (109.934, -38.5983)
  point P1 (189.4728, -90.2737)
  dimension "d307" = 3
  dimension "d308" = 3
  dimension "d309" = 3
  dimension "d310" = 3
  dimension "d311" = 10
  dimension "d312" = 10
  dimension "d313" = 10
  dimension "d314" = 10
  dimension "d317" = 20
  dimension "d318" = 20
  dimension "d328" = 226
  constraints: 8 centre point, 4 concentric, 4 end point, 2 horizontal alignment, 2 vertical alignment, 1 tangent
  measures "d307" diameter of A0
  measures "d308" diameter of A1
  measures "d309" diameter of A2
  measures "d310" diameter of A3
  measures "d311" diameter of A4
  measures "d312" diameter of A5
  measures "d313" diameter of A6
  measures "d314" diameter of A7
  measures "d317" distance from line of L2 A0.centre
  measures "d318" distance from line of L5 A1.centre
  measures "d328" distance of A0.centre A3.centre
extrude "Wyciągnięcie proste59" cut sketch "Szkic85" against normal blind 10 contours A0 | A1 | A2 | A3
ref_plane "Płaszczyzna konstrukcyjna23" through (0, 72, 0) normal (0, 1, 0) x (-1, 0, 0)
sketch "Szkic86" plane through (0, 72, 0) normal (0, 1, 0) x (-1, 0, 0)
  circle A0 centre (-112.9518, 27) radius 1.5 projected
  circle A1 centre (-112.9518, 27) radius 2.5
  line L0 (118.0482, -130) -> (118.0482, 47.011) projected
  line L1 (105.3748, -42.7089) -> (105.3748, 35.3763) projected
  line L2 (105.3748, -130) -> (105.3748, -87.2911) projected
  line L3 (118.0482, -130) -> (105.3748, -130) projected
  circle A2 centre (-113.0482, -110) radius 2.5
  circle A3 centre (113.0482, 27) radius 2.5
  circle A4 centre (113.0482, -110) radius 2.5
  point P0 (0, 0)
  dimension "d322" = 5
  dimension "d323" = 5
  dimension "d324" = 5
  dimension "d325" = 5
  constraints: 4 centre point, 3 coincident, 1 vertical alignment, 5 other
  measures "d322" diameter of A1
  measures "d323" diameter of A2
  measures "d324" diameter of A3
  measures "d325" diameter of A4
extrude "Wyciągnięcie proste60" cut sketch "Szkic86" against normal blind 47.25 contours A0 | A1 | A2 | A3 | A4
